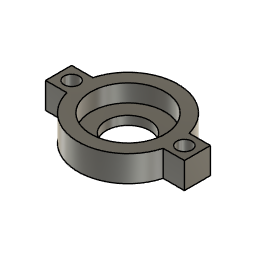
bearing_mount (Autodesk Fusion 360 design; units mm, degrees)
Autodesk Fusion 360 part; units mm, degrees
sketch "Szkic1" plane through (0, 0, 0) normal (0, 0, 1) x (1, 0, 0)
  circle A0 centre (0, 0) radius 5
  circle A1 centre (0, 0) radius 8.5
  circle A2 centre (0, 0) radius 11.5
  circle A3 centre (13, 0) radius 1.75
  circle A4 centre (-13, 0) radius 1.75
  line L0 (16, 3) -> (-16, 3)
  line L1 (-16, 3) -> (-16, -3)
  line L2 (-16, -3) -> (16, -3)
  line L3 (16, -3) -> (16, 3)
  line L4 (16, 3) -> (-16, -3) construction
  line L5 (-16, 3) -> (16, -3) construction
  dimension "d1" = 10
  dimension "d2" = 17
  dimension "d3" = 23
  dimension "d4" = 3.5
  dimension "d5" = 13
  dimension "d6" = 3.5
  dimension "d7" = 13
  dimension "d8" = 32
  dimension "d9" = 6
  constraint coincident A0.centre A1.centre
  constraint concentric A0 A2
  constraint horizontal L0
  constraint perpendicular L0 L1
  constraint parallel L0 L2
  constraint parallel L1 L3
  constraint coincident L4 A0.centre
  constraint coincident L5 A0.centre
  constraint horizontal A0.centre A4.centre
  constraint horizontal A0.centre A3.centre
  measures "d1" diameter of A0
  measures "d2" diameter of A1
  measures "d3" diameter of A2
  measures "d4" diameter of A3
  measures "d5" distance of A0.centre A3.centre
  measures "d6" diameter of A4
  measures "d7" distance of A0.centre A4.centre
  measures "d8" distance of L1.end L2.end
  measures "d9" distance of L0.end L1.end
extrude "Wyciągnięcie proste1" add sketch "Szkic1" along normal blind 6 contours A1 A2 A3 L0 L2 | A1 A2 L0 | A1 A2 L2 | A1 A2 A4 L0 L2 | A2 A3 L0 L2 L3 | A2 A4 L0 L1 L2
extrude "Wyciągnięcie proste2" add sketch "Szkic1" along normal blind 2 contours A0 A1 L0 L2 | A0 A1 L0 | A0 A1 L2 | A0 A1 L0 L2
